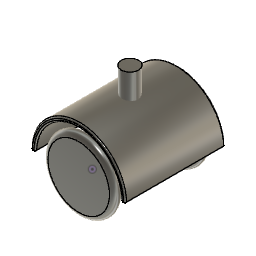
Wheel v8 (Autodesk Fusion 360 design; units mm, degrees)
Autodesk Fusion 360 part; units mm, degrees
sketch "Sketch1" plane through (0, 0, 0) normal (0, 0, 1) x (1, 0, 0)
sketch "Sketch2" plane through (0, 0, 0) normal (0, 1, 0) x (1, 0, 0)
  circle A0 centre (0, 0) radius 10
  dimension "d1" = 20
  constraint coincident A0.centre origin
  measures "d1" diameter of A0
extrude "Extrude1" add sketch "Sketch2" along normal blind 50 makes body 1
sketch "Sketch3" plane through (0, 0, 0) normal (0, -1, 0) x (1, 0, 0)
  circle A0 centre (0, 0) radius 10
  circle A1 centre (0, 0) radius 7.5
  dimension "d4" = 15
  constraint coincident A0.centre A1.centre
  measures "d4" diameter of A1
extrude "Extrude2" cut sketch "Sketch3" against normal blind 145 contours A1 bodies 1
sketch "Sketch4" plane through (0, 0, 0) normal (0, 1, 0) x (1, 0, 0)
sketch "Sketch1 (2)" plane through (0, 0, 0) normal (0, 1, 0) x (1, 0, 0) in component "Component"
  circle A0 centre (0, 0) radius 25
  constraint coincident A0.centre origin
extrude "Extrude1'" add sketch "Sketch1 (2)" against normal blind 7 separate body makes body 2 in component "Component"
fillet "Fillet1" radius 3.5 2 edges at (-23.3082, -7, -9.0404) (-23.3082, 0, 9.0404) on bodies 2 in component "Component"
copy_body "CopyPasteBodies1" bodies 2 makes body 3
move_body "Move1" bodies 3 to x (1, 0, 0) y (0, 1, 0) z (0, 0, 1) at (0, 130, 0)
move_body "Align1" bodies 3 to x (1, 0, 0) y (0, 1, 0) z (0, 0, 1) at (0, -73, 0)
sketch "Sketch1 (3)" plane through (0, 0, 0) normal (0, 1, 0) x (1, 0, 0) in component "Component'"
  circle A0 centre (0, 0) radius 6
  dimension "d12" = 12
  constraint coincident A0.centre origin
  measures "d12" diameter of A0
extrude "Extrude1''" add sketch "Sketch1 (3)" along normal blind 55 separate body makes body 4 in component "Component'"
move_body "Move2" bodies 3 to x (1, 0, 0) y (0, 1, 0) z (0, 0, 1) at (0, 50, 0)
copy_body "Body->Comp1" bodies 3 removing the originals makes body 5 in component "Component''"
ref_plane "WorkPlane1" through (0, 0, 50) normal (0, 0, 1) x (1, 0, 0)
sketch "Sketch6" plane through (0, 0, 50) normal (0, 0, 1) x (1, 0, 0)
  circle A0 centre (0.1118, 26.2789) radius 6
  dimension "d25" = 12
  measures "d25" diameter of A0
extrude "Extrude3" add sketch "Sketch6" along normal up to surface end surface at (9.9503, 16.6667, 0.9957) on bodies 1 bodies 1
ref_plane "WorkPlane2" through (0, 60, 0) normal (0, 1, 0) x (0, 0, 1)
sketch "Sketch7" plane through (0, 60, 0) normal (0, 1, 0) x (1, 0, 0)
  arc A0 (-30, 0) -> (30, 0) centre (0, 0) ccw
  constraint coincident A0.centre origin
surface "Extrude4" add extruded along (0, 1, 0) between 0 and -70 path "Sketch7" along A0 separate body makes body 6
thicken "Thicken1" add thickness 3 1 faces at (23.914, 36.6667, 18.1141) separate body on bodies 6 makes body 7
fillet "Fillet1'" radius 1 2 edges at (0, 60, 33) (0, 60, 30) on bodies 7
fillet "Fillet2" radius 1 2 edges at (0, -10, 33) (0, -10, 30) on bodies 7
fillet "Fillet3" radius 1 8 edges at (32.7071, -9.7071, 0) (31.5, -10, 0) (30.2929, -9.7071, 0) (30, 25, 0) (30.2929, 59.7071, 0) (31.5, 60, 0) (32.7071, 59.7071, 0) (33, 25, 0) on bodies 7
fillet "Fillet4" radius 1 8 edges at (-31.5, -10, 0) (-30.2929, -9.7071, 0) (-30, 25, 0) (-30.2929, 59.7071, 0) (-31.5, 60, 0) (-32.7071, 59.7071, 0) (-33, 25, 0) (-32.7071, -9.7071, 0) on bodies 7
extrude "Extrude5" add 1 faces at (9.1015, 50, 0.8694) along direction (0, 1, 0) up to surface (2.5 mm away) on bodies 1 bodies 1
component "Component" placed x (1, 0, 0) y (0, 1, 0) z (0, 0, 1) at (0, -2.5, 0)
component "Component'" placed x (1, 0, 0) y (0, 1, 0) z (0, 0, 1) at (0, -2.5, 0)
component "Component''" placed x (1, 0, 0) y (0, 1, 0) z (0, 0, 1) at (0, -47.5, 0)
hidden bodies 6
